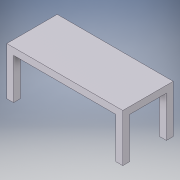
# Autodesk Inventor part: computerBottom
Saved by Autodesk Inventor 2017 (Build 210142000, 142)
## iProperties
Created: 2018-09-10
Part Number: computerBottom
Material: Aluminum 6061, Welded
Document SubType Name: Modeling
Designer: emmacarlisle
Density: 2.7 g/cm^3
Appearance: Weld - Aluminum
Author: emmacarlisle
Autodesk Inventor part; units mm, degrees
ref_plane "YZ Plane" through (0, 0, 0) normal (1, 0, 0) x (0, 1, 0)
ref_plane "XZ Plane" through (0, 0, 0) normal (0, 1, 0) x (-1, 0, 0)
ref_plane "XY Plane" through (0, 0, 0) normal (0, 0, 1) x (1, 0, 0)
sketch "Sketch1" plane through (0, 0, 0) normal (0, 0, 1) x (1, 0, 0)
  point P0 (0, 0)
sketch "Sketch2" plane through (0, 0, 0) normal (0, 0, 1) x (1, 0, 0)
  line L0 (0, 0) -> (1700, 0)
  line L1 (1700, 0) -> (1700, 700)
  line L2 (1700, 700) -> (0, 700)
  line L3 (0, 700) -> (0, 0)
  dimension "d0" = 700
  dimension "d1" = 1700
  constraints: 8 end point, 2 parallel, 1 coincident, 1 horizontal, 1 perpendicular
  measures "d0" distance of L2.end L0.start
  measures "d1" distance of L1.end L2.end
extrude "Extrusion1" add sketch "Sketch2" along normal blind 740
sketch "Sketch3" plane through (0, 0, 740) normal (0, 0, 1) x (1, 0, 0)
  line L0 (1600, 0) -> (100, 0)
  line L1 (100, 0) -> (100, 600)
  line L2 (100, 600) -> (1600, 600)
  line L3 (1600, 600) -> (1600, 0)
  line L4 (1700, 700) -> (0, 700) projected
  line L5 (1700, 0) -> (1700, 700) projected
  line L6 (0, 700) -> (0, 0) projected
  dimension "d4" = 100
  dimension "d5" = 100
  dimension "d6" = 100
  constraints: 8 end point, 2 parallel, 1 horizontal, 1 perpendicular
  measures "d4" distance between parallel lines of L4 L2
  measures "d5" distance between parallel lines of L5 L3
  measures "d6" distance between parallel lines of L6 L1
extrude "Extrusion2" cut sketch "Sketch3" against normal blind 740
sketch "Sketch4" plane through (1700, 0, 0) normal (1, 0, 0) x (0, 0, -1)
  line L0 (0, 0) -> (-740, 0) projected
  line L1 (-640, 0) -> (-100, 0)
  line L2 (-100, 0) -> (-100, 600)
  line L3 (-100, 600) -> (-640, 600)
  line L4 (-640, 600) -> (-640, 0)
  line L5 (0, 700) -> (-740, 700) projected
  line L6 (-740, 600) -> (-740, 0) projected
  line L7 (0, 0) -> (0, 700) projected
  dimension "d9" = 100
  dimension "d10" = 100
  dimension "d11" = 100
  constraints: 8 end point, 2 parallel, 1 horizontal, 1 perpendicular, 1 point on line
  measures "d9" distance between parallel lines of L5 L3
  measures "d10" distance between parallel lines of L6 L4
  measures "d11" distance between parallel lines of L7 L2
extrude "Extrusion3" cut sketch "Sketch4" against normal blind 4000
body "Solid1"
